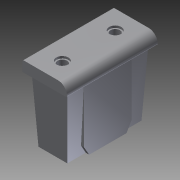
# Autodesk Inventor part: 1XXX.500_Montageblocke
Saved by Autodesk Inventor 2016 (Build 200138000, 138)
## iProperties
Category: PARTsolutions
Company: RITTAL
Created: 2014-04-04
Part Number: 1XXX.500_Montageblocke
Catalog Web Link: www.cadenas.de
Description: Montageblöcke AE-Montageblöcke AE
Vendor: RITTAL
Document SubType Name: Modeling
Designer: PARTuser1
Manufacturer: RITTAL
Density: 1 g/cm^3
Material: Generic
Appearance: RGB(175.00000476837209,175.00000476837209,175.00000476837209)
PSOL_IDENT_0: {$CADENAS_DATA\23d-libs\rittal\schaltschranksys\kompakt_schaltschr\ae\parts_ae\montageblocke_ae.prj}
PSOL_IDENT_1: ,196 {VTYP=3D},{NB=1XXX.500_Montageblocke},{LINA=1XXX.500_Montageblocke},{NN=Montageblöcke AE},{DATE
PSOL_IDENT_2: =27.03.2014 09:06:31},{GEOMDATE=27.03.2014 09:06:00},{VERSION=},{LINEID=10},{LINESUBID=-1},{WBVAR=}
PSOL_IDENT_3: {NB=1XXX.500_Montageblocke},{LINA=1XXX.500_Montageblocke},{KT=DUMMY},{BEST=1XXX.500},{VERS=1},{D=13
PSOL_IDENT_4: 3.000},{E=43.000}
CNS_NN: Montageblöcke AE
CNS_NT: Montageblöcke AE
CNS_NB: 1XXX.500_Montageblocke
CNS_NBSYN: $BEST._Montageblocke
CNS_LINA: 1XXX.500_Montageblocke
CNS_BEST: 1XXX.500
CNS_VERS: 1
CNS_D: 133.000
CNS_E: 43.000
SUPPLIER: RITTAL
ARTICLENO: 1XXX.500_Montageblocke
BOMINFO: 1XXX.500_Montageblocke
CREATOR: CADENAS GmbH
Title: 1XXX.500_Montageblocke
Author: Cadenas PARTsolutions
Comments: Montageblöcke AE
Autodesk Inventor part; units mm, degrees
sketch "Sketch_1" plane through (0, 0, 0) normal (0, 1, 0) x (-1, 0, 0)
  line L0 (5.5, 0) -> (-6.3, 0)
  line L1 (-6.3, 0) -> (-5.1732, -21.5)
  line L2 (-5.1732, -21.5) -> (4.3732, -21.5)
  line L3 (4.3732, -21.5) -> (5.5, 0)
  constraints: 8 end point
extrude "Extrusion1" add sketch "Sketch_1" along normal mid plane 26.8
sketch "Sketch_2" plane through (0, 0, 0) normal (1, 0, 0) x (0, 1, 0)
  line L0 (13.4, 0) -> (12.2732, -21.5)
  line L1 (12.2732, -21.5) -> (-12.2732, -21.5)
  line L2 (-12.2732, -21.5) -> (-13.4, 0)
  line L3 (-13.4, 0) -> (-15, 0)
  line L4 (-15, 0) -> (-15, -25)
  line L5 (-15, -25) -> (15, -25)
  line L6 (15, -25) -> (15, 0)
  line L7 (15, 0) -> (13.4, 0)
  constraints: 16 end point
extrude "Extrusion2" cut sketch "Sketch_2" along normal mid plane 13
sketch "Sketch_3" plane through (-7, 0, 0) normal (1, 0, 0) x (0, 0, -1)
  line L0 (0, -7.9) -> (18.5, -7.9)
  line L1 (18.5, -7.9) -> (21.5, -6.1679)
  line L2 (21.5, -6.1679) -> (21.5, 6.1679)
  line L3 (21.5, 6.1679) -> (18.5, 7.9)
  line L4 (18.5, 7.9) -> (0, 7.9)
  line L5 (0, 7.9) -> (0, -7.9)
  constraints: 12 end point
extrude "Extrusion3" add sketch "Sketch_3" along normal blind 13.3
sketch "Sketch_4" plane through (0, 0, 0) normal (0, 1, 0) x (-1, 0, 0)
  line L0 (7, 0) -> (7, 3)
  arc A0 (7, 3) -> (6.5, 3.5) centre (6.5, 3) ccw
  line L1 (6.5, 3.5) -> (-4.8, 3.5)
  arc A1 (-4.8, 3.5) -> (-7.8, 0.5) centre (-4.8, 0.5) ccw
  arc A2 (-7.8, 0.5) -> (-7.3, 0) centre (-7.3, 0.5) ccw
  line L2 (-7.3, 0) -> (7, 0)
  constraints: 6 end point, 6 point on circle, 3 centre point
extrude "Extrusion4" add sketch "Sketch_4" along normal mid plane 30
sketch "Sketch5" plane through (-6.5, 15, 3.5) normal (0, 0, 1) x (1, 0, 0)
  point P0 (6.5, -6.25)
hole "Drilling 1" at (0, 8.75, 3.5) direction (0, 0, -1) diameter 3.1 depth 11.2 tip angle 120 counterbore diameter 4 counterbore depth 0.7
sketch "Sketch6" plane through (-6.5, 15, 3.5) normal (0, 0, 1) x (1, 0, 0)
  point P0 (6.5, -23.75)
hole "Drilling 2" at (0, -8.75, 3.5) direction (0, 0, -1) diameter 3.1 depth 11.2 tip angle 120 counterbore diameter 4 counterbore depth 0.7
sketch "Sketch7" plane through (5.1732, 12.2732, -21.5) normal (0, 0, -1) x (-1, 0, 0)
  point P0 (5.1732, -6.0232)
hole "Drilling 3" at (0, 6.25, -21.5) direction (0, 0, 1) diameter 3.1 depth 10 tip angle 120 counterbore diameter 4 counterbore depth 1.5
sketch "Sketch8" plane through (5.1732, 12.2732, -21.5) normal (0, 0, -1) x (-1, 0, 0)
  point P0 (5.1732, -18.5232)
hole "Drilling 4" at (0, -6.25, -21.5) direction (0, 0, 1) diameter 3.1 depth 10 tip angle 120 counterbore diameter 4 counterbore depth 1.5
sketch "Sketch9" plane through (-7, 0, 0) normal (-1, 0, 0) x (0, 0, 1)
  point P0 (-15, 0)
hole "Drilling 5" at (-7, 0, -15) direction (1, 0, 0) diameter 3.1 depth 11 tip angle 120 counterbore diameter 4 counterbore depth 1.5
ref_plane "montageblocke_XY" through (0, -8.75, 3.5) normal (0, 0, 1) x (1, 0, 0)
ref_plane "montageblocke_YZ" through (0, -8.75, 3.5) normal (1, 0, 0) x (0, 1, 0)
ref_plane "montageblocke_ZX" through (0, -8.75, 3.5) normal (0, 1, 0) x (0, 0, 1)
ref_plane "montageblocke_2_XY" through (0, 8.75, 3.5) normal (0, 0, 1) x (1, 0, 0)
ref_plane "montageblocke_2_YZ" through (0, 8.75, 3.5) normal (1, 0, 0) x (0, 1, 0)
ref_plane "montageblocke_2_ZX" through (0, 8.75, 3.5) normal (0, 1, 0) x (0, 0, 1)
body "Solid1"
